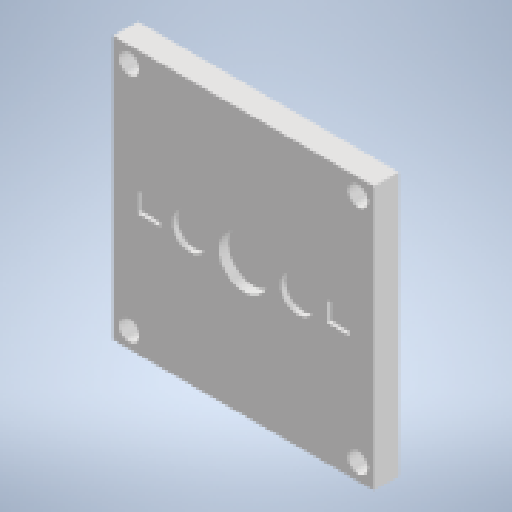
# Autodesk Inventor part: parte superior
Saved by Autodesk Inventor 2024 (Build 280153000, 153)
## iProperties
Created: 2023-07-04
Part Number: parte superior
Material: Generic
Document SubType Name: Modeling
Designer: Kleber
Density: 1 g/cm^3
Appearance: Default
Author: Kleber
Autodesk Inventor part; units mm, degrees
ref_plane "YZ Plane" through (0, 0, 0) normal (1, 0, 0) x (0, 1, 0)
ref_plane "XZ Plane" through (0, 0, 0) normal (0, 1, 0) x (-1, 0, 0)
ref_plane "XY Plane" through (0, 0, 0) normal (0, 0, 1) x (1, 0, 0)
sketch "Sketch1" plane through (0, 0, 0) normal (0, 0, 1) x (1, 0, 0)
  line L0 (52.5, 53) -> (52.5, -53) projected
  line L1 (-52.5, 53) -> (52.5, 53) projected
  line L2 (52.5, 53) -> (-52.5, 53)
  line L3 (-52.5, 53) -> (-52.5, -53)
  line L4 (-52.5, -53) -> (52.5, -53)
  line L5 (52.5, -53) -> (52.5, 53)
  line L6 (50.5, -51) -> (50.5, 51) projected
  line L7 (50.5, 51) -> (-50.5, 51) projected
  line L8 (50.5, 51) -> (-50.5, 51)
  line L9 (-50.5, 51) -> (-50.5, -51)
  line L10 (-50.5, -51) -> (50.5, -51)
  line L11 (50.5, -51) -> (50.5, 51)
  point P0 (0, 0)
  constraints: 16 end point, 4 parallel, 2 horizontal, 2 perpendicular
extrude "Extrusion1" add sketch "Sketch1" along normal blind 10
sketch "Sketch2" plane through (0, 0, 0) normal (0, 0, -1) x (-1, 0, 0)
  circle A0 centre (-46, 46.5) radius 1.5 projected
  line L0 (-50.5, 51) -> (-50.5, 42) projected
  line L1 (-41.5, 51) -> (-50.5, 51) projected
  line L2 (-41.5, 51) -> (-41.5, 42) projected
  line L3 (-41.5, 42) -> (-50.5, 42) projected
  circle A1 centre (-46, -46.5) radius 1.5 projected
  line L4 (-41.5, -42) -> (-41.5, -51) projected
  line L5 (-50.5, -51) -> (-41.5, -51) projected
  line L6 (-50.5, -42) -> (-50.5, -51) projected
  line L7 (-50.5, -42) -> (-41.5, -42) projected
  circle A2 centre (46, -46.5) radius 1.5 projected
  line L8 (50.5, -51) -> (50.5, -42) projected
  line L9 (41.5, -51) -> (50.5, -51) projected
  line L10 (41.5, -51) -> (41.5, -42) projected
  line L11 (41.5, -42) -> (50.5, -42) projected
  circle A3 centre (46, 46.5) radius 1.5 projected
  line L12 (41.5, 42) -> (41.5, 51) projected
  line L13 (50.5, 51) -> (41.5, 51) projected
  line L14 (50.5, 42) -> (50.5, 51) projected
  line L15 (50.5, 42) -> (41.5, 42) projected
  point P0 (0, 0)
extrude "Extrusion2" add sketch "Sketch2" against normal blind 10
sketch "Sketch3" plane through (0, 0, 10) normal (0, 0, 1) x (1, 0, 0)
  line L0 (43.467, -7.68) -> (39.533, -7.68) projected
  line L1 (39.533, -7.68) -> (39.533, -6.68) projected
  line L2 (39.533, -6.68) -> (43.467, -6.68) projected
  line L3 (43.467, -6.68) -> (43.467, -7.68) projected
  line L4 (41.5, 42) -> (41.5, 51) projected
  line L5 (41.5, 51) -> (-41.5, 51) projected
  line L6 (-41.5, 51) -> (-41.5, 42) projected
  line L7 (-41.5, 42) -> (-50.5, 42) projected
  line L8 (-50.5, 42) -> (-50.5, -42) projected
  line L9 (-50.5, -42) -> (-41.5, -42) projected
  line L10 (-41.5, -42) -> (-41.5, -51) projected
  line L11 (-41.5, -51) -> (41.5, -51) projected
  line L12 (41.5, -51) -> (41.5, -42) projected
  line L13 (41.5, -42) -> (50.5, -42) projected
  line L14 (50.5, -42) -> (50.5, 42) projected
  line L15 (50.5, 42) -> (41.5, 42) projected
  line L16 (43.467, -7.68) -> (39.533, -7.68) projected
  line L17 (39.533, -7.68) -> (39.533, -6.68) projected
  line L18 (39.533, -6.68) -> (43.467, -6.68) projected
  line L19 (43.467, -6.68) -> (43.467, -7.68) projected
  line L20 (41.5, 42) -> (41.5, 51) projected
  line L21 (41.5, 51) -> (-41.5, 51) projected
  line L22 (-41.5, 51) -> (-41.5, 42) projected
  line L23 (-41.5, 42) -> (-50.5, 42) projected
  line L24 (-50.5, 42) -> (-50.5, -42) projected
  line L25 (-50.5, -42) -> (-41.5, -42) projected
  line L26 (-41.5, -42) -> (-41.5, -51) projected
  line L27 (-41.5, -51) -> (41.5, -51) projected
  line L28 (41.5, -51) -> (41.5, -42) projected
  line L29 (41.5, -42) -> (50.5, -42) projected
  line L30 (50.5, -42) -> (50.5, 42) projected
  line L31 (50.5, 42) -> (41.5, 42) projected
  circle A0 centre (44.2752, 10.8885) radius 1.8923 projected
  circle A1 centre (-22.2674, 46.7091) radius 1.9651 projected
  line L32 (38.467, -7.68) -> (34.533, -7.68) projected
  line L33 (34.533, -7.68) -> (34.533, -6.68) projected
  line L34 (34.533, -6.68) -> (38.467, -6.68) projected
  line L35 (38.467, -6.68) -> (38.467, -7.68) projected
  circle A2 centre (-36.634, 10.3057) radius 1.9118 projected
  circle A3 centre (44.2752, 10.8885) radius 1.8923 projected
  circle A4 centre (-22.2674, 46.7091) radius 1.9651 projected
  line L36 (38.467, -7.68) -> (34.533, -7.68) projected
  line L37 (34.533, -7.68) -> (34.533, -6.68) projected
  line L38 (34.533, -6.68) -> (38.467, -6.68) projected
  line L39 (38.467, -6.68) -> (38.467, -7.68) projected
  circle A5 centre (-36.634, 10.3057) radius 1.9118 projected
  point P0 (0, 0)
extrude "Extrusion3" add sketch "Sketch3" against normal blind 5 contours L0 L1 L2 L3 | L15 L14 L13 L12 L11 L10 L9 L8 L7 L6 L5 L4 | A0 | A1 | L32 L33 L34 L35 | A2
sketch "Sketch4" plane through (0, 0, 10) normal (0, 0, 1) x (1, 0, 0)
  circle A0 centre (46, 46.5) radius 1.5 projected
  circle A1 centre (46, -46.5) radius 1.5 projected
  circle A2 centre (-46, -46.5) radius 1.5 projected
  circle A3 centre (-46, 46.5) radius 1.5 projected
  circle A4 centre (46, 46.5) radius 4
  circle A5 centre (46, -46.5) radius 4
  circle A6 centre (-46, -46.5) radius 4
  circle A7 centre (-46, 46.5) radius 4
  point P0 (0, 0)
  dimension "d6" = 8
  dimension "d7" = 8
  dimension "d8" = 8
  dimension "d9" = 8
  constraints: 4 centre point, 4 coincident
  measures "d6" diameter of A4
  measures "d7" diameter of A5
  measures "d8" diameter of A6
  measures "d9" diameter of A7
extrude "Extrusion4" cut sketch "Sketch4" against normal blind 8
sketch "Sketch5" plane through (0, 0, 10) normal (0, 0, 1) x (1, 0, 0)
  line L0 (-52.5, -53) -> (52.5, -53) projected
  line L1 (52.5, -53) -> (52.5, 53) projected
  line L2 (-52.5, -53) -> (52.5, -53)
  line L3 (52.5, -53) -> (52.5, 53)
  line L4 (52.5, 53) -> (-52.5, 53)
  line L5 (-52.5, 53) -> (-52.5, -53)
  line L6 (-52.5, 53) -> (-52.5, 0)
  circle A0 centre (0, 0) radius 10
  line L7 (-52.5, 0) -> (-42.5, 0)
  line L8 (-42.5, 0) -> (-42.5, 4)
  line L9 (-42.5, 4) -> (-33.5, 4)
  line L10 (-33.5, 4) -> (-33.5, -4)
  line L11 (-33.5, -4) -> (-42.5, -4)
  line L12 (-42.5, -4) -> (-42.5, 0)
  line L13 (-33.5, 0) -> (-10, 0)
  line L14 (-10, 0) -> (-21.75, 0)
  circle A1 centre (-21.75, 0) radius 7
  line L15 (0, 0) -> (21.75, 0)
  line L16 (42.5, 0) -> (42.5, -4)
  line L17 (42.5, -4) -> (33.5, -4)
  line L18 (33.5, -4) -> (33.5, 4)
  line L19 (33.5, 4) -> (42.5, 4)
  line L20 (42.5, 4) -> (42.5, 0)
  circle A2 centre (21.75, 0) radius 7
  point P0 (33.5, 0)
  dimension "d12" = 20
  dimension "d14" = 10
  dimension "d15" = 4
  dimension "d16" = 9
  dimension "d17" = 8
  dimension "d18" = 14
  dimension "d19" = 21.75
  dimension "d20" = 4
  dimension "d21" = 9
  dimension "d22" = 8
  dimension "d23" = 14
  constraints: 38 end point, 9 perpendicular, 4 midpoint, 3 coincident, 3 parallel, 3 point on line, 2 centre point, 2 horizontal, 1 horizontal alignment, 2 other
  measures "d14" distance of L6.end L7.end
  measures "d15" distance of L7.end L8.end
  measures "d16" distance of L8.end L9.end
  measures "d17" distance of L9.end L10.end
  measures "d18" diameter of A1
  measures "d19" distance of L15.start L15.end
  measures "d20" distance of L20.end L17.start
  measures "d21" distance of L17.start L18.start
  measures "d22" distance of L18.start L18.end
  measures "d23" diameter of A2
extrude "Extrusion5" cut sketch "Sketch5" against normal blind 4 contours A0
extrude "Extrusion6" cut sketch "Sketch5" against normal blind 2.2 contours A2 | A1 L13 | L13 A1
extrude "Extrusion7" cut sketch "Sketch5" against normal blind 1.5 contours L8 L9 L10 L11 L12 | L16 L17 L18 L19 L20
sketch "Sketch6" plane through (0, 0, 0) normal (0, 0, -1) x (-1, 0, 0)
  line L0 (-41.5, 42) -> (-41.5, 51) projected
  line L1 (-50.5, 42) -> (-41.5, 42) projected
  line L2 (-50.5, -42) -> (-50.5, 42) projected
  line L3 (-41.5, -42) -> (-50.5, -42) projected
  line L4 (-41.5, -51) -> (-41.5, -42) projected
  line L5 (41.5, -51) -> (-41.5, -51) projected
  line L6 (41.5, -42) -> (41.5, -51) projected
  line L7 (50.5, -42) -> (41.5, -42) projected
  line L8 (50.5, 42) -> (50.5, -42) projected
  line L9 (41.5, 42) -> (50.5, 42) projected
  line L10 (41.5, 51) -> (41.5, 42) projected
  line L11 (-41.5, 51) -> (41.5, 51) projected
  circle A0 centre (-46, 46.5) radius 1.5 projected
  circle A1 centre (-46, -46.5) radius 1.5 projected
  circle A2 centre (46, -46.5) radius 1.5 projected
  circle A3 centre (46, 46.5) radius 1.5 projected
  line L12 (-52.5, -53) -> (-52.5, 53) projected
  line L13 (52.5, -53) -> (-52.5, -53) projected
  line L14 (52.5, 53) -> (52.5, -53) projected
  line L15 (-52.5, 53) -> (52.5, 53) projected
  line L16 (-50.5, 42) -> (-50.5, -42) projected
  line L17 (-50.5, 42) -> (-41.5, 42) projected
  line L18 (-41.5, 42) -> (-41.5, 51) projected
  line L19 (41.5, 51) -> (-41.5, 51) projected
  line L20 (41.5, 51) -> (41.5, 42) projected
  line L21 (41.5, 42) -> (50.5, 42) projected
  line L22 (50.5, -42) -> (50.5, 42) projected
  line L23 (50.5, -42) -> (41.5, -42) projected
  line L24 (41.5, -42) -> (41.5, -51) projected
  line L25 (-41.5, -51) -> (41.5, -51) projected
  line L26 (-41.5, -51) -> (-41.5, -42) projected
  line L27 (-41.5, -42) -> (-50.5, -42) projected
  line L28 (41.5, -51) -> (50.5, -51)
  line L29 (50.5, -51) -> (50.5, -42)
  line L30 (-41.5, -51) -> (-50.5, -51)
  line L31 (-50.5, -51) -> (-50.5, -42)
  line L32 (-50.5, 42) -> (-50.5, 51)
  line L33 (-50.5, 51) -> (-41.5, 51)
  line L34 (50.5, 42) -> (50.5, 51)
  line L35 (50.5, 51) -> (41.5, 51)
  point P0 (0, 0)
  constraints: 16 end point, 5 perpendicular, 2 horizontal, 2 point on line
extrude "Extrusion8" add sketch "Sketch6" along normal blind 0.5 contours L1 L32 L33 L0 | L35 L34 L9 L10 | L3 L4 L30 L31 | L29 L28 L6 L7
body "Solid1"
